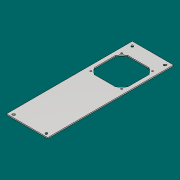
# Autodesk Inventor part: bottom_panel
Saved by Autodesk Inventor 2018.2 (Build 222227000, 227)
## iProperties
Created: 2019-10-14
Part Number: bottom_panel
Material: アルミニウム 6061
Document SubType Name: Modeling
Designer: gisen
Density: 2.7 g/cm^3
Appearance: アルミニウム - フラット
Author: gisen
Autodesk Inventor part; units mm, degrees
ref_plane "YZ Plane" through (0, 0, 0) normal (1, 0, 0) x (0, 1, 0)
ref_plane "XZ Plane" through (0, 0, 0) normal (0, 1, 0) x (-1, 0, 0)
ref_plane "XY Plane" through (0, 0, 0) normal (0, 0, 1) x (1, 0, 0)
sketch "スケッチ1" plane through (0, 0, 0) normal (0, 0, 1) x (1, 0, 0)
  line L0 (-55, -170) -> (55, -170)
  line L1 (55, -170) -> (55, 170)
  line L2 (55, 170) -> (-55, 170)
  line L3 (-55, 170) -> (-55, -170)
  line L4 (-55, -170) -> (55, 170) construction
  line L5 (55, -170) -> (-55, 170) construction
  line L6 (-55, 140) -> (-50, 140) construction
  line L7 (-50, 140) -> (-25, 165) construction
  line L8 (-25, 165) -> (-25, 170) construction
  line L9 (-46, 40.5) -> (46, 40.5) construction
  line L10 (46, 40.5) -> (46, 132.5) construction
  line L11 (46, 132.5) -> (-46, 132.5) construction
  line L12 (-46, 132.5) -> (-46, 40.5) construction
  line L13 (-46, 40.5) -> (46, 132.5) construction
  line L14 (46, 40.5) -> (-46, 132.5) construction
  line L15 (-46, 1.5) -> (46, 1.5) construction
  line L16 (46, 1.5) -> (46, 37.5) construction
  line L17 (46, 37.5) -> (-46, 37.5) construction
  line L18 (-46, 37.5) -> (-46, 1.5) construction
  line L19 (-46, 1.5) -> (46, 37.5) construction
  line L20 (46, 1.5) -> (-46, 37.5) construction
  line L21 (0, 0) -> (0, 86.5) construction
  circle A0 centre (0, 86.5) radius 53 construction
  line L22 (-44.7, 41.8) -> (44.7, 41.8) construction
  line L23 (44.7, 41.8) -> (44.7, 131.2) construction
  line L24 (44.7, 131.2) -> (-44.7, 131.2) construction
  line L25 (-44.7, 131.2) -> (-44.7, 41.8) construction
  line L26 (-44.7, 41.8) -> (44.7, 131.2) construction
  line L27 (44.7, 41.8) -> (-44.7, 131.2) construction
  arc A1 (-28.4765, 131.2) -> (-44.7, 114.9765) centre (0, 86.5) ccw
  arc A2 (-44.7, 58.0235) -> (-28.4765, 41.8) centre (0, 86.5) ccw
  arc A3 (28.4765, 41.8) -> (44.7, 58.0235) centre (0, 86.5) ccw
  arc A4 (44.7, 114.9765) -> (28.4765, 131.2) centre (0, 86.5) ccw
  line L28 (-28.4765, 131.2) -> (28.4765, 131.2)
  line L29 (-44.7, 114.9765) -> (-44.7, 58.0235)
  line L30 (-28.4765, 41.8) -> (28.4765, 41.8)
  line L31 (44.7, 58.0235) -> (44.7, 114.9765)
  line L32 (-41.25, 45.25) -> (41.25, 45.25) construction
  line L33 (41.25, 45.25) -> (41.25, 127.75) construction
  line L34 (41.25, 127.75) -> (-41.25, 127.75) construction
  line L35 (-41.25, 127.75) -> (-41.25, 45.25) construction
  line L36 (-41.25, 45.25) -> (41.25, 127.75) construction
  line L37 (41.25, 45.25) -> (-41.25, 127.75) construction
  circle A5 centre (-41.25, 127.75) radius 2.25
  circle A6 centre (-41.25, 45.25) radius 2.25
  circle A7 centre (41.25, 45.25) radius 2.25
  circle A8 centre (41.25, 127.75) radius 2.25
  circle A9 centre (-45, 160) radius 2.25
  circle A10 centre (45, 160) radius 2.25
  circle A11 centre (45, -160) radius 2.25
  circle A12 centre (-45, -160) radius 2.25
  circle A13 centre (-45, 0) radius 2.25 construction
  circle A14 centre (45, 0) radius 2.25 construction
  line L38 (-55, 0) -> (55, 0) construction
  circle A15 centre (-41.25, -49.75) radius 2.25
  arc A16 (-44.7, -36.9765) -> (-28.4765, -53.2) centre (0, -8.5) ccw
  line L39 (-28.4765, -53.2) -> (28.4765, -53.2)
  arc A17 (28.4765, -53.2) -> (44.7, -36.9765) centre (0, -8.5) ccw
  circle A18 centre (41.25, -49.75) radius 2.25
  line L40 (44.7, -36.9765) -> (44.7, 19.9765)
  circle A19 centre (41.25, 32.75) radius 2.25
  arc A20 (44.7, 19.9765) -> (28.4765, 36.2) centre (0, -8.5) ccw
  line L41 (-28.4765, 36.2) -> (28.4765, 36.2)
  circle A21 centre (-41.25, 32.75) radius 2.25
  arc A22 (-28.4765, 36.2) -> (-44.7, 19.9765) centre (0, -8.5) ccw
  line L42 (-44.7, 19.9765) -> (-44.7, -36.9765)
  circle A23 centre (-41.25, -144.75) radius 2.25
  arc A24 (-44.7, -131.9765) -> (-28.4765, -148.2) centre (0, -103.5) ccw
  line L43 (-28.4765, -148.2) -> (28.4765, -148.2)
  arc A25 (28.4765, -148.2) -> (44.7, -131.9765) centre (0, -103.5) ccw
  circle A26 centre (41.25, -144.75) radius 2.25
  line L44 (44.7, -131.9765) -> (44.7, -75.0235)
  circle A27 centre (41.25, -62.25) radius 2.25
  arc A28 (44.7, -75.0235) -> (28.4765, -58.8) centre (0, -103.5) ccw
  line L45 (-28.4765, -58.8) -> (28.4765, -58.8)
  circle A29 centre (-41.25, -62.25) radius 2.25
  arc A30 (-28.4765, -58.8) -> (-44.7, -75.0235) centre (0, -103.5) ccw
  line L46 (-44.7, -75.0235) -> (-44.7, -131.9765)
  point P0 (0, 19.5)
  point P1 (0, 19.5)
  dimension "d12" = 106
  dimension "d0" = 110
  dimension "d1" = 340
  dimension "d2" = 135
  dimension "d3" = 30
  dimension "d4" = 30
  dimension "d5" = 5
  dimension "d6" = 92
  dimension "d7" = 92
  dimension "d8" = 92
  dimension "d9" = 36
  dimension "d10" = 3
  dimension "d11" = 1.5
  dimension "d13" = 89.4
  dimension "d14" = 89.4
  dimension "d15" = 82.5
  dimension "d16" = 82.5
  dimension "d17" = 4.5
  dimension "d25" = 4.5
  dimension "d26" = 10
  dimension "d27" = 10
  dimension "d28" = 10
  dimension "d29" = 10
  dimension "d30" = 10
  dimension "d31" = 10
  dimension "d32" = 10
  dimension "d33" = 10
  dimension "d34" = 10
  dimension "d35" = 10
  dimension "d45" = 95
  constraints: 94 end point, 30 centre point, 24 point on circle, 15 coincident, 13 midpoint, 13 point on line, 10 parallel, 8 equal radius, 8 perpendicular, 6 horizontal, 2 vertical, 1 collinear, 66 other
  measures "d0" distance of L2.end L1.end
  measures "d1" distance of L1.end L0.end
  measures "d2" angle of L7 L6
  measures "d3" distance between parallel lines of L8 L3
  measures "d4" distance between parallel lines of L2 L6
  measures "d5" distance of L7.end L8.end
  measures "d6" distance of L11.end L10.end
  measures "d7" distance of L10.end L9.end
  measures "d8" distance of L17.end L16.end
  measures "d9" distance of L16.end L15.end
  measures "d10" distance between parallel lines of L17 L9
  measures "d11" distance from line of L21.start L15
  measures "d13" distance of L24.end L23.end
  measures "d14" distance of L23.end L22.end
  measures "d15" distance of L34.end L33.end
  measures "d16" distance of L33.end L32.end
  measures "d17" diameter of A5
  measures "d25" diameter of A9
  measures "d26" distance from line of A9.centre L2
  measures "d27" distance from line of L3 A9.centre
  measures "d28" distance from line of L2 A10.centre
  measures "d29" distance from line of L1 A10.centre
  measures "d30" distance from line of L1 A11.centre
  measures "d31" distance from line of L0 A11.centre
  measures "d32" distance from line of L0 A12.centre
  measures "d33" distance from line of L3 A12.centre
  measures "d34" distance from line of L3 A13.centre
  measures "d35" distance from line of L1 A14.centre
  measures "d45" distance of A6.centre A15.centre
extrude "押し出し1" add sketch "スケッチ1" along normal blind 3 contours L3 L2 L1 L0 | A15 | L42 A22 L41 A20 L40 A17 L39 A16 | A18 | A19 | A21 | A23 | L46 A30 L45 A28 L44 A25 L43 A24 | A26 | A27 | A29
sketch "スケッチ2" plane through (0, 0, 3) normal (0, 0, 1) x (1, 0, 0)
  circle A0 centre (-45, 160) radius 2.25 construction
  circle A1 centre (45, -160) radius 2.25 construction
  circle A2 centre (-45, -160) radius 2.25 construction
  circle A3 centre (-43, 158) radius 2.75 construction
  line L0 (55, 170) -> (-55, 170) projected
  line L1 (-55, 170) -> (-55, -170) projected
  line L2 (-43.7153, 161.8472) -> (-41.4298, 160.2577)
  line L3 (-45.2577, 156.4298) -> (-46.8472, 158.7153)
  circle A4 centre (-45, 160) radius 2.25 construction
  arc A5 (-43.7153, 161.8472) -> (-46.8472, 158.7153) centre (-45, 160) ccw
  arc A6 (-45.2577, 156.4298) -> (-41.4298, 160.2577) centre (-43, 158) ccw
  line L4 (55, 170) -> (-55, 170) construction
  line L5 (0, 170) -> (0, -170) construction
  line L6 (-55, -170) -> (55, -170) construction
  line L7 (-55, 0) -> (55, 0) construction
  line L8 (55, -170) -> (55, 170) construction
  circle A7 centre (45, 160) radius 2.25 construction
  circle A8 centre (43, 158) radius 2.75 construction
  line L9 (43.7153, 161.8472) -> (41.4298, 160.2577)
  line L10 (45.2577, 156.4298) -> (46.8472, 158.7153)
  circle A9 centre (45, 160) radius 2.25 construction
  arc A10 (46.8472, 158.7153) -> (43.7153, 161.8472) centre (45, 160) ccw
  arc A11 (41.4298, 160.2577) -> (45.2577, 156.4298) centre (43, 158) ccw
  circle A12 centre (-45, -160) radius 2.25 construction
  circle A13 centre (-43, -158) radius 2.75 construction
  line L11 (-43.7153, -161.8472) -> (-41.4298, -160.2577)
  line L12 (-45.2577, -156.4298) -> (-46.8472, -158.7153)
  circle A14 centre (-45, -160) radius 2.25 construction
  arc A15 (-46.8472, -158.7153) -> (-43.7153, -161.8472) centre (-45, -160) ccw
  arc A16 (-41.4298, -160.2577) -> (-45.2577, -156.4298) centre (-43, -158) ccw
  circle A17 centre (45, -160) radius 2.25 construction
  line L13 (45.2577, -156.4298) -> (46.8472, -158.7153)
  arc A18 (45.2577, -156.4298) -> (41.4298, -160.2577) centre (43, -158) ccw
  circle A19 centre (43, -158) radius 2.75 construction
  line L14 (43.7153, -161.8472) -> (41.4298, -160.2577)
  circle A20 centre (45, -160) radius 2.25 construction
  arc A21 (43.7153, -161.8472) -> (46.8472, -158.7153) centre (45, -160) ccw
  point P0 (0, 0)
  dimension "d38" = 5.5
  dimension "d39" = 12
  dimension "d40" = 12
  constraints: 28 point on circle, 27 symmetric about line, 20 end point, 15 centre point, 8 coincident, 4 midpoint, 2 horizontal, 2 tangent, 1 vertical, 25 other
  measures "d38" diameter of A3
  measures "d39" distance from line of A3.centre L0
  measures "d40" distance from line of L1 A3.centre
extrude "押し出し2" cut sketch "スケッチ2" against normal through all
sketch "スケッチ3" plane through (0, 0, 3) normal (0, 0, 1) x (1, 0, 0)
  line L0 (-55, -170) -> (55, -170) construction
  line L1 (-55, -166.5) -> (55, -166.5)
  line L2 (55, -166.5) -> (55, -170)
  line L3 (55, -170) -> (-55, -170)
  line L4 (-55, -170) -> (-55, -166.5)
  line L5 (-55, -166.5) -> (55, -170) construction
  line L6 (55, -166.5) -> (-55, -170) construction
  line L7 (0, -168.25) -> (0, -170) construction
  point P0 (0, 0)
  dimension "d50" = 3.5
  dimension "d51" = 110
  constraints: 14 end point, 4 midpoint, 2 parallel, 1 horizontal, 1 perpendicular, 1 point on line
  measures "d50" distance of L1.end L2.end
  measures "d51" distance of L1.start L1.end
extrude "押し出し3" cut sketch "スケッチ3" against normal through all
sketch "スケッチ4" plane through (0, 0, 3) normal (0, 0, 1) x (1, 0, 0)
  line L0 (-55, -166.5) -> (55, -166.5) construction
  line L1 (55, -166.5) -> (55, 170) construction
  line L2 (55, 170) -> (-55, 170) construction
  line L3 (-55, 170) -> (-55, -166.5) construction
  circle A0 centre (-41.25, 127.75) radius 2.25 construction
  circle A1 centre (-41.25, 45.25) radius 2.25 construction
  circle A2 centre (41.25, 45.25) radius 2.25 construction
  circle A3 centre (41.25, 127.75) radius 2.25 construction
  line L4 (43.7153, -161.8472) -> (41.4298, -160.2577) construction
  arc A4 (45.2577, -156.4298) -> (41.4298, -160.2577) centre (43, -158) ccw construction
  line L5 (45.2577, -156.4298) -> (46.8472, -158.7153) construction
  arc A5 (43.7153, -161.8472) -> (46.8472, -158.7153) centre (45, -160) ccw construction
  line L6 (-28.4765, 131.2) -> (28.4765, 131.2) construction
  arc A6 (44.7, 114.9765) -> (28.4765, 131.2) centre (0, 86.5) ccw construction
  line L7 (44.7, 114.9765) -> (44.7, 58.0235) construction
  arc A7 (28.4765, 41.8) -> (44.7, 58.0235) centre (0, 86.5) ccw construction
  line L8 (28.4765, 41.8) -> (-28.4765, 41.8) construction
  arc A8 (-44.7, 58.0235) -> (-28.4765, 41.8) centre (0, 86.5) ccw construction
  line L9 (-44.7, 58.0235) -> (-44.7, 114.9765) construction
  arc A9 (-28.4765, 131.2) -> (-44.7, 114.9765) centre (0, 86.5) ccw construction
  line L10 (41.4298, 160.2577) -> (43.7153, 161.8472) construction
  arc A10 (46.8472, 158.7153) -> (43.7153, 161.8472) centre (45, 160) ccw construction
  line L11 (46.8472, 158.7153) -> (45.2577, 156.4298) construction
  arc A11 (41.4298, 160.2577) -> (45.2577, 156.4298) centre (43, 158) ccw construction
  line L12 (-45.2577, 156.4298) -> (-46.8472, 158.7153) construction
  arc A12 (-43.7153, 161.8472) -> (-46.8472, 158.7153) centre (-45, 160) ccw construction
  line L13 (-43.7153, 161.8472) -> (-41.4298, 160.2577) construction
  arc A13 (-45.2577, 156.4298) -> (-41.4298, 160.2577) centre (-43, 158) ccw construction
  line L14 (-41.4298, -160.2577) -> (-43.7153, -161.8472) construction
  arc A14 (-46.8472, -158.7153) -> (-43.7153, -161.8472) centre (-45, -160) ccw construction
  line L15 (-46.8472, -158.7153) -> (-45.2577, -156.4298) construction
  arc A15 (-41.4298, -160.2577) -> (-45.2577, -156.4298) centre (-43, -158) ccw construction
  line L16 (-54.75, -166.25) -> (54.75, -166.25)
  line L17 (54.75, -166.25) -> (54.75, 169.75)
  line L18 (54.75, 169.75) -> (-54.75, 169.75)
  line L19 (-54.75, 169.75) -> (-54.75, -166.25)
  point P0 (0, 0)
  dimension "d54" = 0.25
  constraints: 8 end point, 3 other
  measures "d54" distance between parallel lines of L3 L19
extrude "押し出し4" [suppressed]
equation "\"d4\" = d3"
equation "\"d11\" = 0.5 * d10"
equation "\"d27\" = d26"
equation "\"d28\" = d26"
equation "\"d29\" = d26"
equation "\"d30\" = d26"
equation "\"d31\" = d26"
equation "\"d32\" = d26"
equation "\"d33\" = d26"
equation "\"d34\" = d26"
equation "\"d35\" = d26"
equation "\"d45\" = d7 + d10"
